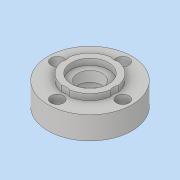
# Autodesk Inventor part: bearingHousing
Saved by Autodesk Inventor 2017 (Build 210142000, 142)
## iProperties
Created: 2016-10-29
Part Number: bearingHousing
Material: Generic
Document SubType Name: Modeling
Designer: techn
Density: 1 g/cm^3
Appearance: Default
Author: techn
Autodesk Inventor part; units mm, degrees
ref_plane "YZ Plane" through (0, 0, 0) normal (1, 0, 0) x (0, 1, 0)
ref_plane "XZ Plane" through (0, 0, 0) normal (0, 1, 0) x (-1, 0, 0)
ref_plane "XY Plane" through (0, 0, 0) normal (0, 0, 1) x (1, 0, 0)
sketch "Sketch1" plane through (0, 0, 0) normal (0, 1, 0) x (-1, 0, 0)
  circle A0 centre (0, 0) radius 5.715
  circle A1 centre (0, 0) radius 3
  circle A2 centre (0, 0) radius 10.16
  line L0 (0, 0) -> (7.9375, 0)
  circle A3 centre (7.9375, 0) radius 1.524
  circle A4 centre (7.9375, 0) radius 2.2225
  circle A5 centre (0, 7.9375) radius 2.2225
  circle A6 centre (0, 7.9375) radius 1.524
  circle A7 centre (-7.9375, 0) radius 2.2225
  circle A8 centre (-7.9375, 0) radius 1.524
  circle A9 centre (0, -7.9375) radius 2.2225
  circle A10 centre (0, -7.9375) radius 1.524
  dimension "d2" = 11.43
  dimension "d3" = 6
  dimension "d4" = 20.32
  dimension "d5" = 7.9375
  dimension "d6" = 3.048
  dimension "d9" = 360
  constraints: 11 centre point, 7 coincident, 2 end point, 1 horizontal, 17 other
  measures "d2" diameter of A0
  measures "d3" diameter of A1
  measures "d4" diameter of A2
  measures "d5" distance of L0.start L0.end
  measures "d6" diameter of A3
extrude "Extrusion1" add sketch "Sketch1" along normal blind 3 contours A4 A2 A9 A0 | A0 A5 A2 A4 | A4 | A0 A7 A2 A5 | A5 | A9 A2 A7 A0 | A9 | A7
sketch "Sketch2" plane through (0, 3, 0) normal (0, 1, 0) x (1, 0, 0)
  circle A0 centre (0, 0) radius 3 projected
  circle A1 centre (0, 7.9375) radius 1.524 projected
  circle A2 centre (7.9375, 0) radius 1.524 projected
  circle A3 centre (0, -7.9375) radius 1.524 projected
  circle A4 centre (-7.9375, 0) radius 1.524 projected
  circle A5 centre (0, 0) radius 5.715 projected
  circle A6 centre (0, 0) radius 10.16 projected
extrude "Extrusion2" add sketch "Sketch2" along normal blind 2.5 contours A5 | A6
sketch "Sketch4" plane through (0, 5.5, 0) normal (0, 1, 0) x (1, 0, 0)
  circle A0 centre (0, 0) radius 4.5
  circle A1 centre (0, 0) radius 6
  dimension "d19" = 9
  dimension "d20" = 12
  constraints: 2 centre point, 2 coincident
  measures "d19" diameter of A0
  measures "d20" diameter of A1
extrude "Extrusion3" add sketch "Sketch4" along normal blind 1.5
sketch "Sketch5" plane through (0, 5.5, 0) normal (0, 1, 0) x (1, 0, 0)
  circle A0 centre (-7.9375, 0) radius 1.524 projected
  circle A1 centre (-7.9375, 0) radius 2.2225
  circle A2 centre (0, -7.9375) radius 2.2225
  circle A3 centre (7.9375, 0) radius 2.2225
  circle A4 centre (0, 7.9375) radius 2.2225
  point P0 (0, 0)
  dimension "d23" = 4.445
  dimension "d26" = 360
  constraints: 4 centre point, 1 coincident, 9 other
  measures "d23" diameter of A1
extrude "Extrusion4" cut sketch "Sketch5" along normal blind 1.5
body "Solid1"
